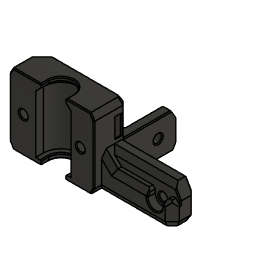
z_bearing_holder_a_x2 (Autodesk Fusion 360 design; units mm, degrees)
Autodesk Fusion 360 part; units mm, degrees
note: some values were not read from the file. Chosen so that the rebuilt part matches the saved one: the sign of a taper; which pieces of a blend or face edit are solid. Set by a fixed rule: which sketch regions a step uses.
sketch "Sketch1" plane through (0, 0, 0) normal (0, 0, 1) x (1, 0, 0)
  circle A0 centre (0, 0) radius 7.5
  line L0 (17.2, 9) -> (47.2, 9)
  line L1 (47.2, 9) -> (47.2, 31.5)
  line L2 (47.2, 31.5) -> (17.2, 31.5)
  line L3 (17.2, 31.5) -> (17.2, 9)
  line L4 (11.7, 31.5) -> (11.7, 10.6)
  line L5 (8.2, 31.5) -> (8.2, 10.6)
  line L6 (17.2, 31.5) -> (8.2, 31.5)
  line L7 (47.2, 9) -> (47.2, 0)
  line L8 (17.2, 9) -> (17.2, 4.2018)
  line L9 (17.2, 3.5) -> (47.2, 3.5)
  line L10 (-18.65, -10.6) -> (17.2, -10.6)
  line L11 (-18.65, -10.6) -> (-18.65, 10.6)
  line L12 (17.2, 4.2018) -> (17.2, -10.6)
  line L13 (-12.825, -10.6) -> (-12.825, 8.4) construction
  line L14 (-10, 6) -> (-15.65, 6)
  line L15 (-15.65, 6) -> (-15.65, 8.4)
  line L16 (-15.65, 8.4) -> (-10, 8.4)
  line L17 (-10, 8.4) -> (-10, 6)
  line L18 (-10, 6) -> (-15.65, 8.4) construction
  line L19 (-15.65, 6) -> (-10, 8.4) construction
  line L20 (0, 0) -> (0, 7.5)
  line L21 (-18.65, 10.6) -> (8.2, 10.6)
  line L22 (-18.65, 0) -> (17.2, 0)
  line L23 (47.2, 0) -> (17.2, 0)
  line L24 (8.2, 10.6) -> (17.2, 10.6)
  line L25 (15.65, 6) -> (15.65, 8.4)
  line L26 (15.65, 8.4) -> (10, 8.4)
  line L27 (10, 8.4) -> (10, 6)
  line L28 (10, 6) -> (15.65, 6)
  line L29 (-0.95, 10.6) -> (8.2, 19.75)
  line L30 (8.2, 19.75) -> (17.2, 19.75)
  circle A1 centre (0, 0) radius 5.25
  line L31 (17.2, 24) -> (32.2, 9)
  line L32 (-7.5, 0) -> (-7.5, -10.6)
  line L33 (7.5, 0) -> (7.5, -10.6)
  line L34 (-5.25, -3.25) -> (-18.65, -3.25)
  line L35 (5.25, -3.25) -> (17.2, -3.25)
  line L36 (-5.25, 0) -> (-5.25, -3.25)
  line L37 (5.25, 0) -> (5.25, -3.25)
  point P0 (-12.825, 7.2)
  dimension "d1" = 15
  dimension "d3" = 30
  dimension "d4" = 22.5
  dimension "d5" = 5.5
  dimension "d8" = 3.5
  dimension "d9" = 5.5
  dimension "d11" = 10.6
  dimension "d13" = 19
  dimension "d14" = 5.65
  dimension "d15" = 2.4
  dimension "d16" = 3
  dimension "d17" = 10.6
  dimension "d19" = 17.2
  dimension "d20" = 3.5
  dimension "d21" = 10
  dimension "d22" = 45
  dimension "d23" = 9.15
  dimension "d24" = 10.5
  dimension "d42" = 45
  dimension "d43" = 15
  dimension "d45" = 3.25
  constraint coincident A0.centre L20.start
  constraint horizontal L0
  constraint vertical L1
  constraint horizontal L2
  constraint vertical L3
  constraint vertical L4
  constraint vertical L5
  constraint horizontal L6
  constraint coincident L5.start L6.end
  constraint vertical L7
  constraint coincident L8.end L3
  constraint coincident L8 L9.start
  constraint coincident L7 L9.end
  constraint horizontal L9
  constraint vertical L11
  constraint horizontal L10
  constraint vertical L12
  constraint coincident L10.end L12.end
  constraint coincident L10 L13.start
  constraint perpendicular L10 L13
  constraint horizontal L14
  constraint perpendicular L14 L15
  constraint parallel L14 L16
  constraint parallel L15 L17
  constraint coincident L18 P0
  constraint coincident L19 P0
  constraint coincident A0 L20.end
  constraint midpoint L13.end L16
  constraint coincident L5 L21.end
  constraint horizontal L21
  constraint coincident L11 L22.start
  constraint coincident L12 L22.end
  constraint horizontal L22
  constraint horizontal L23
  constraint coincident L22.end L23.end
  constraint coincident L4.start L6
  constraint coincident L3 L24.end
  constraint coincident L4.end L24
  constraint symmetric L14.start L20 L27.end
  constraint symmetric L14.end L20 L25.start
  constraint symmetric L15.end L20 L25.end
  constraint symmetric L16.end L20 L26.end
  constraint vertical L20
  constraint coincident A0.centre L22
  constraint coincident L21 L29.start
  constraint coincident L5 L29.end
  constraint horizontal L24
  constraint coincident L3 L30.end
  constraint horizontal L30
  constraint concentric A0 A1
  constraint coincident L3 L31.start
  constraint coincident L0 L31.end
  constraint coincident L22 L32.start
  constraint coincident A0 L32.start
  constraint coincident L10 L32.end
  constraint tangent A0 L32
  constraint coincident L22 L33.start
  constraint coincident A0 L33.start
  constraint coincident L10 L33.end
  constraint tangent A0 L33
  constraint coincident L11 L34.end
  constraint horizontal L34
  constraint coincident L12 L35.end
  constraint horizontal L35
  constraint collinear L34 L35
  constraint coincident A1 L36.start
  constraint coincident L22 L36.start
  constraint vertical L36
  constraint coincident L34.start L36.end
  constraint coincident L22 L37.start
  constraint coincident A1 L37.start
  constraint coincident L35.start L37.end
  constraint vertical L37
  measures "d1" diameter of A0
  measures "d3" distance of L0.start L0.end
  measures "d4" distance of L0.start L2.end
  measures "d5" distance of L3 L4
  measures "d8" distance of L4 L5
  measures "d9" distance of L0 L9
  measures "d11" distance of A0.centre L10
  measures "d13" distance of L13.start L13.end
  measures "d14" distance of L15.end L16.end
  measures "d15" distance of L14.end L15.end
  measures "d16" distance of L11 L15
  measures "d17" distance of A0.centre L21
  measures "d19" distance of A0.centre L12
  measures "d20" distance of L9 L23
  measures "d21" distance of A0.centre L17
  measures "d22" angle of L5 L29
  measures "d23" distance of L21 L29.end
  measures "d24" diameter of A1
  measures "d42" angle of L0 L31
  measures "d43" distance of L0.start L31.end
  measures "d45" distance of L22 L34
extrude "Extrude2" add sketch "Sketch1" along normal blind 15 contours A0 L3 L8 L11 L12 L21 L22 L24 | L12 L22 L33 L35 | L11 L22 L32 L34 | L0 L7 L8 L9 L12 | L3 L4 L24 L30 | L3 L4 L6 L30 | L14 L15 L16 L17 | L25 L26 L27 L28
extrude "Extrude3" add sketch "Sketch1" along normal blind 10 contours L7 L9 L12 L23 | L5 L21 L29 | L4 L5 L24 L30 | L4 L5 L6 L30
extrude "Extrude5" add sketch "Sketch1" along normal blind 26.5 contours A0 L3 L8 L11 L12 L21 L22 L24 | L12 L22 L33 L35 | L11 L22 L32 L34 | L14 L15 L16 L17 | L25 L26 L27 L28
extrude "Extrude6" add sketch "Sketch1" along normal blind 2 contours A0 L20 L22 A1 | A0 L33 L35 | A0 L22 L35 L37 | A0 L3 L8 L11 L12 L21 L22 L24 | L12 L22 L33 L35 | A0 L20 L22 A1 | L7 L9 L12 L23 | A0 L22 L34 L36 | L11 L22 L32 L34 | A0 L32 L34 | L0 L7 L8 L9 L12 | L5 L21 L29 | L3 L4 L24 L30 | L4 L5 L24 L30 | L4 L5 L6 L30 | L3 L4 L6 L30 | L14 L15 L16 L17 | L25 L26 L27 L28
extrude "Extrude7" add sketch "Sketch1" along normal blind 3.5 from surface at 26.5 contours A0 L20 L22 A1 | A0 L33 L35 | A0 L22 L35 L37 | A0 L3 L8 L11 L12 L21 L22 L24 | L12 L22 L33 L35 | A0 L20 L22 A1 | A0 L22 L34 L36 | L11 L22 L32 L34 | A0 L32 L34 | L14 L15 L16 L17 | L25 L26 L27 L28
chamfer "Chamfer2" distance 2.15 angle 45 1 edges at (0, 5.25, 26.5)
chamfer "Chamfer5" distance 5 angle 45 1 edges at (17.2, 1.75, 10)
sketch "Sketch2" plane through (17.2, 0, 0) normal (1, 0, 0) x (0, 1, 0)
  line L0 (31.5, 0) -> (31.5, 15)
  line L1 (3.5, 15) -> (9, 15)
  line L2 (10.6, 15) -> (10.6, 30)
  line L3 (10.6, 30) -> (-3.25, 30)
  line L4 (-3.25, 30) -> (-3.25, 0)
  line L5 (-3.25, 0) -> (0, 0)
  line L6 (0, 0) -> (0, 15)
  line L7 (9, 15) -> (9, 0)
  line L8 (9, 0) -> (31.5, 0)
  circle A0 centre (24, 7.5) radius 1.75
  circle A1 centre (24, 7.5) radius 3.25
  line L9 (27.25, 7.5) -> (27.25, 15)
  line L10 (20.75, 7.5) -> (20.75, 15)
  line L11 (0, 15) -> (3.5, 15)
  line L12 (31.5, 15) -> (10.6, 15)
  dimension "d46" = 3.5
  dimension "d47" = 6.5
  dimension "d48" = 7.5
  dimension "d49" = 7.5
  constraint concentric A0 A1
  constraint coincident A1 L9.start
  constraint tangent A1 L9
  constraint coincident L1 L9.end
  constraint perpendicular L1 L9
  constraint coincident A1 L10.start
  constraint tangent A1 L10
  constraint coincident L1 L10.end
  constraint perpendicular L1 L10
  measures "d46" diameter of A0
  measures "d47" diameter of A1
  measures "d48" distance of L0 A0.centre
  measures "d49" distance of L8 A0.centre
extrude "Extrude8" cut sketch "Sketch2" against normal blind 9 contours A0
extrude "Extrude9" cut sketch "Sketch2" against normal blind 35 from surface at -5.5 contours A1 L9 L10 L12 | A1 | A0
sketch "Sketch3" plane through (0, 9, 0) normal (0, 1, 0) x (-1, 0, 0)
  line L0 (-17.2, 0) -> (-17.2, 15)
  line L1 (-17.2, 15) -> (-47.2, 15)
  line L2 (-47.2, 15) -> (-47.2, 0)
  line L3 (-47.2, 0) -> (-17.2, 0)
  circle A0 centre (-39.7, 7.5) radius 1.75
  circle A1 centre (-39.7, 7.5) radius 3.25
  line L4 (-36.45, 7.5) -> (-36.45, 15)
  line L5 (-42.95, 7.5) -> (-42.95, 15)
  dimension "d56" = 3.5
  dimension "d57" = 6.5
  dimension "d58" = 7.5
  dimension "d59" = 7.5
  constraint concentric A0 A1
  constraint coincident A1 L4.start
  constraint tangent A1 L4
  constraint coincident L1 L4.end
  constraint perpendicular L1 L4
  constraint coincident A1 L5.start
  constraint tangent A1 L5
  constraint coincident L1 L5.end
  constraint perpendicular L1 L5
  measures "d56" diameter of A0
  measures "d57" diameter of A1
  measures "d58" distance of L2 A0.centre
  measures "d59" distance of L3 A0.centre
extrude "Extrude10" cut sketch "Sketch3" against normal blind 9 contours A0
extrude "Extrude11" cut sketch "Sketch3" against normal blind 3.5 from surface at -5.5 contours L1 A1 L4 L5 | A1
sketch "Sketch4" plane through (0, 10.6, 0) normal (0, 1, 0) x (-1, 0, 0)
  line L0 (18.65, 0) -> (18.65, 30)
  line L1 (18.65, 30) -> (-17.2, 30)
  line L2 (-17.2, 30) -> (-17.2, 15)
  line L3 (-17.2, 15) -> (-11.7, 15)
  line L4 (-11.7, 15) -> (-11.7, 10)
  line L5 (-11.7, 10) -> (0.95, 10)
  line L6 (0.95, 10) -> (0.95, 0)
  line L7 (0.95, 0) -> (18.65, 0)
  line L8 (0.725, 30) -> (0.725, 0)
  line L9 (15.65, 12.175) -> (10, 12.175)
  line L10 (10, 12.175) -> (10, 17.825)
  line L11 (10, 17.825) -> (15.65, 17.825)
  line L12 (15.65, 17.825) -> (15.65, 12.175) construction
  line L13 (15.65, 12.175) -> (10, 17.825) construction
  line L14 (10, 12.175) -> (15.65, 17.825) construction
  circle A0 centre (12.825, 15) radius 1.75
  line L15 (18.65, 0) -> (-8.2, 0)
  circle A1 centre (-11.375, 15) radius 1.75
  line L16 (15.65, 17.825) -> (18.65, 17.825)
  line L17 (15.65, 12.175) -> (18.65, 12.175)
  line L18 (-17.2, 15) -> (-17.2, 12.175)
  line L19 (-7.3798, 15) -> (-11.375, 18.9952)
  line L20 (-11.375, 18.9952) -> (-15.3702, 15) construction
  line L21 (-15.3702, 15) -> (-11.375, 11.0048)
  line L22 (-11.375, 11.0048) -> (-7.3798, 15)
  line L23 (-7.3798, 15) -> (-15.3702, 15) construction
  line L24 (-11.375, 18.9952) -> (-11.375, 11.0048) construction
  line L25 (-11.375, 18.9952) -> (-17.2, 24.8202)
  line L26 (-15.3702, 15) -> (-17.2, 16.8298)
  point P0 (12.825, 15)
  point P1 (-11.375, 15)
  dimension "d126" = 5.65
  dimension "d127" = 5.65
  dimension "d128" = 3.5
  dimension "d129" = 5.825
  dimension "d130" = 15
  dimension "d131" = 5.65
  dimension "d132" = 5.65
  constraint midpoint L1 L8.start
  constraint vertical L8
  constraint coincident L7 L8.end
  constraint horizontal L9
  constraint perpendicular L9 L10
  constraint parallel L9 L11
  constraint parallel L10 L12
  constraint coincident L13 P0
  constraint coincident L14 P0
  constraint coincident P0 A0.centre
  constraint symmetric L8 A0 A1
  constraint coincident L0 L16.end
  constraint perpendicular L0 L16
  constraint coincident L0 L17.end
  constraint perpendicular L0 L17
  constraint symmetric L8 L17.end L18.end
  constraint coincident L2.end L3.start
  constraint perpendicular L19 L20
  constraint parallel L19 L21
  constraint parallel L20 L22
  constraint coincident L23 P1
  constraint coincident L24 P1
  constraint coincident P1 A1.centre
  constraint horizontal L23
  constraint coincident L2 L25.end
  constraint perpendicular L20 L25
  constraint coincident L2 L26.end
  constraint perpendicular L20 L26
  measures "d126" distance of L10.end L11.end
  measures "d127" distance of L9.end L10.end
  measures "d128" diameter of A0
  measures "d129" distance of L0 P0
  measures "d130" distance of P0 L15
  measures "d131" distance of L20.end L21.end
  measures "d132" distance of L19.end L20.end
extrude "Extrude12" cut sketch "Sketch4" against normal blind 2.4 from surface at -2.2 contours L0 L9 L10 L11 L16 L17 | L3 L4 A1 L21 | L2 L3 L4 A1 L19 L21 L22 L25 L26 | L3 L4 A1 | L3 L4 A1 | A0
extrude "Extrude13" cut sketch "Sketch4" against normal blind 12.15 from surface at -1.7 contours L3 L4 A1 | L3 L4 A1 | A0
draft "Draft1" angle 45 neutral plane through (0, 8.4, 0) pull (0, -1, 0) 1 faces at (9.6337, 8.7333, 15.1742)
draft "Draft2" angle -45 neutral plane through (0, 8.4, 0) pull (0, 1, 0) 1 faces at (-14.5663, 8.7333, 14.8258)
chamfer "Chamfer6" distance 2 angle 45 3 edges at (45.075, 0, 10) (29.325, 0, 10) (19.7, 0, 12.5)
chamfer "Chamfer7" distance 2 angle 45 1 edges at (32.2, 3.5, 15)
chamfer "Chamfer8" distance 1 angle 45 1 edges at (47.2, 9, 7.5)
chamfer "Chamfer9" distance 3 angle 45 1 edges at (47.2, 0, 4)
chamfer "Chamfer10" distance 2 angle 45 1 edges at (47.2, 3.25, 10)
chamfer "Chamfer11" distance 1 angle 45 1 edges at (36.45, 2.75, 10)
chamfer "Chamfer12" distance 1 angle 45 1 edges at (42.95, 2.75, 10)
chamfer "Chamfer13" distance 0.4 angle 45 5 edges at (36.45, 0.5, 8.5) (39.7, 0, 4.25) (36.45, 0, 7.75) (42.95, 0, 7.75) (42.95, 0.5, 8.5)
chamfer "Chamfer14" distance 0.4 angle 45 1 edges at (41.3316, 3.5, 8.1328)
chamfer "Chamfer25" distance 2 angle 45 1 edges at (8.2, 29.375, 10)
chamfer "Chamfer31" distance 0.4 angle 45 4 edges at (8.2, 24, 4.25) (8.2, 27.25, 7.75) (9.2, 27.25, 9) (10.95, 27.25, 10)
chamfer "Chamfer32" distance 0.4 angle 45 1 edges at (11.7, 22.3684, 8.1328)
chamfer "Chamfer33" distance 0.4 angle 45 2 edges at (17.2, 22.3684, 8.1328) (41.3316, 9, 8.1328)
chamfer "Chamfer35" distance 1.5 angle 45 1 edges at (17.2, 10.6, 22.5)
chamfer "Chamfer36" distance 5 angle 45 1 edges at (-18.65, 10.6, 15)
chamfer "Chamfer37" distance 1.5 angle 60 5 edges at (17.2, 2.925, 30) (-18.65, 1.175, 30) (-16.15, 8.1, 30) (1.025, 10.6, 30) (16.45, 9.85, 30) measured on face at (13.1389, 2.4658, 30) measured on face at (13.1389, 2.4658, 30) measured on face at (-16.05, 8.2, 25.9417) measured on face at (13.1389, 2.4658, 30) measured on face at (16.7, 9.6, 25)
chamfer "Chamfer38" distance 1.5 angle 60 11 edges at (17.2, -1.625, 0) (-18.65, 1.175, 0) (-16.15, 8.1, 0) (-7.3, 10.6, 0) (3.625, 15.175, 0) (8.2, 25.625, 0) (12.7, 31.5, 0) (30.7, 0, 0) (45.7, 1.5, 0) (47.2, 5.5, 0) (46.7, 8.5, 0) measured on face at (9.5578, 10.9515, 0) measured on face at (9.5578, 10.9515, 0) measured on face at (-16.05, 8.2, 4.0583) measured on face at (9.5578, 10.9515, 0) measured on face at (9.5578, 10.9515, 0) measured on face at (8.2, 25.3541, 1.3138) measured on face at (11.2, 31.5, 2.6667) measured on face at (9.5578, 10.9515, 0) measured on face at (46.2, 2, 2.6667) measured on face at (9.5578, 10.9515, 0) measured on face at (46.5333, 8.6667, 5)
chamfer "Chamfer39" distance 0.4 angle 45 18 edges at (0, 5.25, 0) (5.25, -1.625, 0) (-5.25, -1.625, 0) (10.475, -3.25, 0) (-11.2, -3.25, 0) (30.6393, 9, 0) (17.2, 19.5, 0) (-17.9, -3.25, 1.299) (-18.65, -3.25, 15) (-17.9, -3.25, 28.701) (-11.2, -3.25, 30) (10.475, -3.25, 30) (0, 5.25, 30) (5.25, -1.625, 30) (-5.25, -1.625, 30) (16.45, -3.25, 28.701) (17.2, -3.25, 15) (16.45, -3.25, 1.299) measured on face at (10.0578, 10.7444, 0) measured on face at (5.25, -1.0833, 0.6667) measured on face at (10.0578, 10.7444, 0) measured on face at (12.0686, -3.25, 5.951) measured on face at (10.0578, 10.7444, 0) measured on face at (10.0578, 10.7444, 0) measured on face at (10.0578, 10.7444, 0) measured on face at (-18.15, 2.4429, 1.7321) measured on face at (-18.65, 2.65, 19.134) measured on face at (-18.15, 2.4429, 28.2679) measured on face at (12.1971, 2.0037, 30) measured on face at (12.1971, 2.0037, 30) measured on face at (12.1971, 2.0037, 30) measured on face at (12.1971, 2.0037, 30) measured on face at (12.1971, 2.0037, 30) measured on face at (16.7, 4.7762, 28.2679) measured on face at (12.0686, -3.25, 5.951) measured on face at (16.2, -0.5833, 0.866)
chamfer "Chamfer40" distance 3 angle 60 1 edges at (47.2, 6.75, 15) measured on face at (36.8667, 6.6667, 15)
chamfer "Chamfer41" distance 0.4 angle 45 3 edges at (45.2, 9, 13.2679) (30.7, 9, 15) (17.2, 20.3, 15) measured on face at (46.5849, 5, 10.8692) measured on face at (26.2, 7.8333, 15) measured on face at (14.8667, 24.5333, 15)
chamfer "Chamfer42" distance 0.4 angle 45 3 edges at (0, 5.25, 2) (5.25, -1.625, 2) (-5.25, -1.625, 2) measured on face at (-6.75, -1.0833, 2) measured on face at (-6.75, -1.0833, 2) measured on face at (-6.75, -1.0833, 2)
chamfer "Chamfer43" distance 0.4 angle 45 2 edges at (46.2774, 3.5, 11.4019) (47.2, 3.5, 8.9019) measured on face at (46.5849, 5, 10.8692) measured on face at (33.3349, 3.5, 12)
chamfer "Chamfer44" distance 2 angle 45 4 edges at (10.15, 20.75, 10) (8.4, 20.55, 10) (8.2, 20.05, 10) (3.625, 15.175, 10) measured on face at (6.3167, 13.65, 10) measured on face at (8.4667, 20.6167, 9.1667) measured on face at (6.3167, 13.65, 10) measured on face at (6.3167, 13.65, 10)
chamfer "Chamfer45" distance 4 angle 45 1 edges at (11.7, 10.6, 12.5) measured on face at (11.7, 20.2833, 13.3333)
chamfer "Chamfer46" distance 2 angle 45 2 edges at (11.7, 23.05, 15) (9.7, 12.6, 15) measured on face at (13.4, 25.8667, 15) measured on face at (9.0333, 11.9333, 11.6667)
chamfer "Chamfer47" distance 1 angle 45 1 edges at (8.2, 31.5, 5.299) measured on face at (12.3667, 31.5, 5.0654)
chamfer "Chamfer48" distance 2 angle 60 1 edges at (15.25, 31.5, 15) measured on face at (15.7667, 18.2572, 15)
chamfer "Chamfer49" distance 0.4 angle 45 4 edges at (11.7, 31.5, 10.7679) (9.7, 31.5, 9.5) (10.95, 31.5, 10) (11.7, 31.0774, 12.2679) measured on face at (12.7, 31.5, 5.0654) measured on face at (8.8667, 28.6, 8.6667) measured on face at (11.2, 28.9333, 10) measured on face at (14.2, 30.5516, 13.1786)
chamfer "Chamfer54" distance 0.4 angle 45 2 edges at (-11.1934, 6, 15.6328) (13.0066, 6, 15.6328)
chamfer "Chamfer55" distance 0.4 angle 45 2 edges at (13.0066, -3.25, 14.3672) (-11.1934, -3.25, 14.3672)
chamfer "Chamfer57" distance 0.4 angle 45 3 edges at (17.2, 7.2, 16.8298) (17.2, 8.4, 20.825) (17.2, 6, 20.825)
chamfer "Chamfer58" distance 0.4 angle 45 1 edges at (-17.05, 7.2, 12.175)
chamfer "Chamfer59" distance 1 angle 45 1 edges at (-15.85, 8.4, 14.8)
equation "d4 = 15 mm + 7.5 mm"
equation "d13 = 16 mm + 3 mm"
equation "d23 = 7.5 mm + 1.65 mm"
equation "d33 = 15 mm + 4.75 mm + 4.75 mm + 2 mm"
equation "d38 = 4.75 mm + 4.75 mm + 2 mm + 15 mm"
